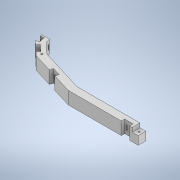
# Autodesk Inventor part: bumper_base_final _원본수정
Saved by Autodesk Inventor 2020 (Build 240168000, 168)
## iProperties
Created: 2022-06-30
Part Number: bumper_base_final _원본수정
Material: 일반
Document SubType Name: Modeling
Designer: samsung
Density: 1 g/cm^3
Appearance: 기본값
Author: samsung
Autodesk Inventor part; units mm, degrees
ref_plane "YZ Plane" through (0, 0, 0) normal (1, 0, 0) x (0, 1, 0)
ref_plane "XZ Plane" through (0, 0, 0) normal (0, 1, 0) x (-1, 0, 0)
ref_plane "XY Plane" through (0, 0, 0) normal (0, 0, 1) x (1, 0, 0)
sketch "스케치1" plane through (0, 0, 0) normal (0, 1, 0) x (-1, 0, 0)
  line L0 (-417.5, 136.0278) -> (167.5, 136.0278)
  arc A0 (156.6099, 73.7155) -> (-406.6899, 73.6783) centre (-125, -531.4722) ccw
  arc A1 (148.4052, 66.4876) -> (-398.3844, 66.4971) centre (-125, -531.4722) ccw
  line L1 (143.8982, 68.5278) -> (-85, 68.5278)
  line L2 (-165, 68.5278) -> (-393.8982, 68.5278)
  line L3 (-125, -531.4722) -> (-125, 1435.9267)
  circle A2 centre (-125, -531.4722) radius 1967.3989
  line L4 (-125, 111.6599) -> (-436.953, 1411.0375)
  line L5 (-125, 111.6599) -> (186.953, 1411.0375)
  line L6 (-417.5444, 28.5399) -> (-406.6899, 73.6783)
  line L7 (-407.5098, 28.5399) -> (-398.3801, 66.5058)
  arc A3 (1441.9544, 38.2515) -> (-1691.7763, 38.7413) centre (-125, -531.4722) ccw
  line L8 (-371.3038, 78.1512) -> (-261.7019, 111.6599)
  line L9 (-261.7019, 111.6599) -> (11.7019, 111.6599)
  line L10 (-316.5029, 94.9056) -> (-320.1581, 106.8613)
  line L11 (-316.5029, 94.9056) -> (-397.3646, 1416.9826)
  line L12 (-316.5029, 94.9056) -> (-988.7616, 1236.1743)
  line L13 (-398.3844, 66.4971) -> (-125, -531.4722)
  line L14 (-407.5098, 28.5399) -> (-405.1717, 38.2627)
  line L15 (-405.1717, 38.2627) -> (-414.6578, 40.5439)
  line L16 (-405.1717, 38.2627) -> (-1671.8283, 684.2501)
  line L17 (-405.1717, 38.2627) -> (-2007.9181, 38.8589)
  line L18 (-405.1717, 38.2627) -> (-402.8337, 47.9856)
  line L19 (-402.8337, 47.9856) -> (-371.3038, 78.1512)
  line L20 (-387.0687, 63.0684) -> (-400.1089, 76.6983)
  line L21 (-387.0687, 63.0684) -> (-1557.9022, 816.656)
  line L22 (-387.0687, 63.0684) -> (-1051.9279, 1203.8846)
  line L23 (-125, -531.4722) -> (-261.7019, 111.6599)
  line L24 (-125, -531.4722) -> (11.7019, 111.6599)
  line L25 (-417.5444, 28.5399) -> (-407.5098, 28.5399)
  line L26 (-125, -531.4722) -> (-371.3038, 78.1512)
  line L27 (-125, -531.4722) -> (121.3038, 78.1512)
  line L28 (11.7019, 111.6599) -> (121.3038, 78.1512)
  line L29 (167.4556, 28.5399) -> (156.6099, 73.7155)
  line L30 (157.5156, 28.5399) -> (148.4052, 66.4876)
  line L31 (121.3038, 78.1512) -> (152.8486, 47.9794)
  line L32 (155.1841, 38.2515) -> (1758.102, 38.2515)
  line L33 (155.1841, 38.2515) -> (164.5823, 40.5079)
  line L34 (157.5156, 28.5399) -> (167.4556, 28.5399)
  line L35 (155.1841, 38.2515) -> (1422.1711, 683.8137)
  line L36 (66.5029, 94.9056) -> (70.1581, 106.8613)
  line L37 (66.5029, 94.9056) -> (738.7616, 1236.1743)
  line L38 (66.5029, 94.9056) -> (147.3646, 1416.9826)
  line L39 (137.0762, 63.0653) -> (150.1137, 76.6961)
  line L40 (137.0762, 63.0653) -> (801.7772, 1203.965)
  line L41 (137.0762, 63.0653) -> (1307.7755, 816.7906)
  line L42 (-125, -531.4722) -> (148.4052, 66.4876)
  line L43 (-259.0118, 93.6599) -> (9.0118, 93.6599)
  line L44 (111.9521, 62.1879) -> (136.5817, 38.6304)
  line L45 (9.0118, 93.6599) -> (111.9521, 62.1879)
  line L46 (-361.9509, 62.1883) -> (-386.641, 38.5664)
  line L47 (-387.0049, 38.256) -> (-387.0101, 38.2515)
  line L48 (-388.9967, 28.5399) -> (-386.569, 38.6353)
  line L49 (-361.9509, 62.1883) -> (-259.0118, 93.6599)
  line L50 (-407.5098, 28.5399) -> (-388.9967, 28.5399)
  line L51 (136.5817, 38.6304) -> (139.0042, 28.5399)
  line L52 (157.5156, 28.5399) -> (139.0042, 28.5399)
  line L53 (-125, 111.6599) -> (-155, 111.6599)
  line L54 (-155, 111.6599) -> (-155, 93.6599)
  line L55 (-155, 93.6599) -> (-125, 93.6599)
  line L56 (-125, 93.6599) -> (-125, 111.6599)
  point P0 (0, 0)
  point P1 (0, 0)
  point P2 (143.8982, 61.5)
  point P3 (-393.8982, 61.5)
  point P4 (-417.5, 21.5)
  point P5 (-165, 0)
  point P6 (-85, 0)
  point P7 (-85, 12.4229)
  point P8 (167.5, 12.4229)
  point P9 (-393.8982, -388.5)
  point P10 (-165, -388.5)
  point P11 (167.5, -327)
  point P12 (-417.5, -327)
  point P13 (-85, -388.5)
  point P14 (143.8982, -388.5)
  point P15 (162, 21.5)
  point P16 (162, 12.4229)
  point P17 (167.5, 21.5)
  point P18 (-125, 0)
  point P19 (-125, 136.0278)
  point P20 (-125, 136.0278)
  point P21 (-125, 93.6599)
  point P22 (-155, 111.6599)
  dimension "d12" = 657.5
  dimension "d13" = 667.5
  dimension "d15" = 585
  dimension "d25" = 1299.8989
  dimension "d30" = 13.5
  dimension "d31" = 13.5
  dimension "d39" = 999.8126
  dimension "d45" = 13.5
  dimension "d46" = 13.5
  dimension "d50" = 10
  dimension "d51" = 13.5
  dimension "d52" = 13.5
  dimension "d53" = 10
  dimension "d54" = 13.5
  dimension "d55" = 13.5
  dimension "d56" = 12
  dimension "d57" = 12
  dimension "d60" = 10
  dimension "d65" = 13.5
  dimension "d66" = 13.5
  dimension "d68" = 13.5
  dimension "d69" = 13.5
  dimension "d70" = 13.5
  dimension "d71" = 13.5
  dimension "d72" = 10
  dimension "d81" = 18
  dimension "d83" = 18
  dimension "d84" = 18
  dimension "d85" = 18
  dimension "d86" = 18
  dimension "d126" = 30
  constraints: 114 end point, 17 point on circle, 14 point on line, 9 parallel, 8 horizontal, 7 perpendicular, 6 midpoint, 3 centre point, 1 coincident, 1 tangent, 18 other
  measures "d12" radius of A1
  measures "d13" radius of A0
  measures "d15" distance of L29.start L6.start
  measures "d30" angle of L4 L3
  measures "d31" angle of L5 L3
  measures "d39" radial gap between concentric circles of A0 A3
  measures "d45" angle of L10 L11
  measures "d46" angle of L12 L10
  measures "d50" distance of L7.start L14.end
  measures "d51" angle of L16 L15
  measures "d52" angle of L17 L15
  measures "d53" distance of L14.end L18.end
  measures "d54" angle of L20 L22
  measures "d55" angle of L20 L21
  measures "d56" angle of L3 L23
  measures "d57" angle of L24 L3
  measures "d60" angle of L26 L23
  measures "d65" angle of L33 L32
  measures "d66" angle of L35 L33
  measures "d68" angle of L37 L36
  measures "d69" angle of L36 L38
  measures "d70" angle of L40 L39
  measures "d71" angle of L41 L39
  measures "d72" angle of L27 L24
  measures "d81" distance between parallel lines of L9 L43
  measures "d83" distance between parallel lines of L31 L44
  measures "d84" distance between parallel lines of L19 L46
  measures "d85" distance between parallel lines of L14 L48
  measures "d86" distance between parallel lines of L30 L51
  measures "d126" distance of L54.end L55.end
extrude "돌출1" add sketch "스케치1" against normal blind 30 contours L9 L24 L43 L3 | L3 L43 L54 L9 | L28 L27 L1 L45 L43 L24 | L44 L45 L1 L27 | L27 L1 L31 L42 L44 | L42 L31 L30 L52 L51 L44 | L31 L1 L27
sketch "스케치2" plane through (-157.5156, -30, 28.5399) normal (-0.9723699, 0, 0.2334454) x (0.2334454, 0, 0.9723699)
  line L0 (4.3214, 30) -> (4.3214, 0) projected
  line L1 (19.9919, 30) -> (56.694, 30) projected
  line L2 (19.9919, 0) -> (0, 0) projected
  line L3 (19.9919, 30) -> (4.9919, 30)
  line L4 (4.9919, 30) -> (4.9919, 0)
  line L5 (4.9919, 0) -> (19.9919, 0)
  line L6 (19.9919, 0) -> (19.9919, 30)
  point P0 (19.9919, 0)
  dimension "d89" = 15
  constraints: 8 end point, 2 parallel, 1 horizontal, 1 perpendicular, 1 point on line
  measures "d89" distance of L5.end L4.end
extrude "돌출2" cut sketch "스케치2" against normal blind 8
sketch "스케치3" plane through (-149.7367, -30, 26.6724) normal (-0.9723699, 0, 0.2334454) x (0.2334454, 0, 0.9723699)
  line L0 (4.9919, 0) -> (4.9919, 30) projected
  line L1 (19.9919, 0) -> (4.9919, 0) projected
  line L2 (19.9919, 30) -> (19.9919, 0) projected
  line L3 (4.9919, 30) -> (19.9919, 30) projected
  line L4 (18.7419, 20.5) -> (16.2419, 20.5)
  line L5 (16.2419, 20.5) -> (16.2419, 9.5)
  line L6 (16.2419, 9.5) -> (18.7419, 9.5)
  line L7 (18.7419, 9.5) -> (18.7419, 20.5)
  line L8 (18.7419, 20.5) -> (16.2419, 9.5) construction
  line L9 (16.2419, 20.5) -> (18.7419, 9.5) construction
  line L10 (6.2419, 20.5) -> (8.7419, 20.5)
  line L11 (8.7419, 20.5) -> (8.7419, 9.5)
  line L12 (8.7419, 9.5) -> (6.2419, 9.5)
  line L13 (6.2419, 9.5) -> (6.2419, 20.5)
  line L14 (6.2419, 20.5) -> (8.7419, 9.5) construction
  line L15 (8.7419, 20.5) -> (6.2419, 9.5) construction
  point P0 (12.4919, 20.5)
  point P1 (12.4919, 30)
  point P2 (19.9919, 15)
  point P3 (17.4919, 15)
  point P4 (7.4919, 15)
  dimension "d94" = 2.5
  dimension "d95" = 2.5
  dimension "d96" = 3.75
  dimension "d97" = 3.75
  dimension "d98" = 9.5
  dimension "d99" = 9.5
  dimension "d100" = 11
  constraints: 24 end point, 6 midpoint, 4 parallel, 2 horizontal, 2 perpendicular, 1 horizontal alignment, 1 vertical alignment
  measures "d94" distance of L6.end L5.end
  measures "d95" distance of L11.end L12.end
  measures "d96" distance from line of point (12.492, 20.5) L5
  measures "d97" distance from line of L11 point (12.492, 20.5)
  measures "d98" distance between parallel lines of L3 L4
  measures "d99" distance between parallel lines of L3 L10
  measures "d100" distance of L10.end L11.end
extrude "돌출3" cut sketch "스케치3" against normal blind 10 contours L7 L6 L5 L4 | L10 L11 L12 L13
sketch "스케치5" plane through (-121.3038, -30, 78.1512) normal (-0.6912048, 0, 0.7226589) x (0.7226589, 0, 0.6912048)
  line L0 (-43.651, 30) -> (0, 30) projected
  line L1 (-43.651, 30) -> (-43.651, 0) projected
  line L2 (0, 0) -> (-43.651, 0) projected
  line L3 (0, 30) -> (0, 0) projected
  line L4 (-38.3577, 0) -> (-4.2758, 0) projected
  line L5 (-31.8255, 30) -> (-11.8255, 30)
  line L6 (-11.8255, 30) -> (-11.8255, 0)
  line L7 (-11.8255, 0) -> (-31.8255, 0)
  line L8 (-31.8255, 0) -> (-31.8255, 30)
  line L9 (-31.8255, 30) -> (-11.8255, 0) construction
  line L10 (-11.8255, 30) -> (-31.8255, 0) construction
  point P0 (33.6428, 30)
  point P1 (-21.8255, 15)
  point P2 (-31.8255, 30)
  point P3 (-31.8255, 0)
  dimension "d107" = 20
  constraints: 12 end point, 2 midpoint, 2 parallel, 1 horizontal, 1 perpendicular, 1 point on line
  measures "d107" distance of L6.end L7.end
extrude "돌출4" cut sketch "스케치5" against normal blind 8 contours L0 L6 L2 L8
sketch "스케치6" plane through (-115.7742, -30, 72.37) normal (-0.6912048, 0, 0.7226589) x (0.7226589, 0, 0.6912048)
  line L0 (-11.8255, 0) -> (-31.8255, 0) projected
  line L1 (-11.8255, 30) -> (-11.8255, 0) projected
  line L2 (-31.8255, 30) -> (-11.8255, 30) projected
  line L3 (-31.8255, 0) -> (-31.8255, 30) projected
  line L4 (-26.8255, 20.5) -> (-16.8255, 9.5) construction
  line L5 (-16.8255, 20.5) -> (-26.8255, 9.5) construction
  line L6 (-15.5755, 20.5) -> (-18.0755, 20.5)
  line L7 (-18.0755, 20.5) -> (-18.0755, 9.5)
  line L8 (-18.0755, 9.5) -> (-15.5755, 9.5)
  line L9 (-15.5755, 9.5) -> (-15.5755, 20.5)
  line L10 (-15.5755, 20.5) -> (-18.0755, 9.5) construction
  line L11 (-18.0755, 20.5) -> (-15.5755, 9.5) construction
  line L12 (-28.0755, 20.5) -> (-25.5755, 20.5)
  line L13 (-25.5755, 20.5) -> (-25.5755, 9.5)
  line L14 (-25.5755, 9.5) -> (-28.0755, 9.5)
  line L15 (-28.0755, 9.5) -> (-28.0755, 20.5)
  line L16 (-28.0755, 20.5) -> (-25.5755, 9.5) construction
  line L17 (-25.5755, 20.5) -> (-28.0755, 9.5) construction
  point P0 (33.6428, 30)
  point P1 (-21.8255, 15)
  point P2 (-16.8255, 15)
  point P3 (-26.8255, 15)
  dimension "d110" = 10
  dimension "d111" = 11
  dimension "d112" = 2.5
  dimension "d113" = 2.5
  constraints: 28 end point, 6 midpoint, 4 parallel, 2 horizontal, 2 perpendicular
  measures "d110" distance of L4.end L5.end
  measures "d111" distance of L5.start L4.end
  measures "d112" distance of L8.end L7.end
  measures "d113" distance of L13.end L14.end
extrude "돌출5" cut sketch "스케치6" against normal blind 10 contours L9 L8 L7 L6 | L12 L13 L14 L15
sketch "스케치7" plane through (-121.3038, -30, 78.1512) normal (-0.2923717, 0, 0.9563048) x (0.9563048, 0, 0.2923717)
  line L0 (0, 30) -> (114.6098, 30) projected
  line L1 (0, 30) -> (0, 0) projected
  line L2 (114.6098, 0) -> (0, 0) projected
  line L3 (114.6098, 30) -> (114.6098, 0) projected
  line L4 (4.2758, 0) -> (111.9197, 0) projected
  line L5 (47.3049, 30) -> (67.3049, 30)
  line L6 (67.3049, 30) -> (67.3049, 0)
  line L7 (67.3049, 0) -> (47.3049, 0)
  line L8 (47.3049, 0) -> (47.3049, 30)
  line L9 (47.3049, 30) -> (67.3049, 0) construction
  line L10 (67.3049, 30) -> (47.3049, 0) construction
  point P0 (93.1542, 30)
  point P1 (57.3049, 15)
  point P2 (47.3049, 30)
  point P3 (47.3049, 0)
  dimension "d116" = 20
  dimension "d117" = 30
  constraints: 12 end point, 2 midpoint, 2 parallel, 1 horizontal, 1 perpendicular, 1 point on line
  measures "d116" distance of L6.end L7.end
  measures "d117" distance of L5.end L6.end
extrude "돌출6" cut sketch "스케치7" against normal blind 8 contours L0 L6 L2 L8
sketch "스케치8" plane through (-118.9649, -30, 70.5008) normal (-0.2923717, 0, 0.9563048) x (0.9563048, 0, 0.2923717)
  line L0 (47.3049, 0) -> (47.3049, 30) projected
  line L1 (67.3049, 0) -> (47.3049, 0) projected
  line L2 (67.3049, 30) -> (67.3049, 0) projected
  line L3 (47.3049, 30) -> (67.3049, 30) projected
  line L4 (52.3049, 20.5) -> (62.3049, 9.5) construction
  line L5 (62.3049, 20.5) -> (52.3049, 9.5) construction
  line L6 (51.0549, 20.5) -> (53.5549, 20.5)
  line L7 (53.5549, 20.5) -> (53.5549, 9.5)
  line L8 (53.5549, 9.5) -> (51.0549, 9.5)
  line L9 (51.0549, 9.5) -> (51.0549, 20.5)
  line L10 (51.0549, 20.5) -> (53.5549, 9.5) construction
  line L11 (53.5549, 20.5) -> (51.0549, 9.5) construction
  line L12 (63.5549, 20.5) -> (61.0549, 20.5)
  line L13 (61.0549, 20.5) -> (61.0549, 9.5)
  line L14 (61.0549, 9.5) -> (63.5549, 9.5)
  line L15 (63.5549, 9.5) -> (63.5549, 20.5)
  line L16 (63.5549, 20.5) -> (61.0549, 9.5) construction
  line L17 (61.0549, 20.5) -> (63.5549, 9.5) construction
  point P0 (93.1542, 30)
  point P1 (57.3049, 15)
  point P2 (52.3049, 15)
  point P3 (62.3049, 15)
  dimension "d120" = 10
  dimension "d121" = 11
  dimension "d122" = 2.5
  dimension "d123" = 2.5
  constraints: 28 end point, 6 midpoint, 4 parallel, 2 horizontal, 2 perpendicular
  measures "d120" distance of L4.end L5.end
  measures "d121" distance of L5.start L4.end
  measures "d122" distance of L7.end L8.end
  measures "d123" distance of L14.end L13.end
extrude "돌출7" cut sketch "스케치8" against normal blind 10 contours L6 L7 L8 L9 | L15 L14 L13 L12
sketch "스케치9" plane through (-11.7019, 0, 111.6599) normal (0, 0, 1) x (1, 0, 0)
  line L0 (0, 0) -> (166.7019, 0) projected
  line L1 (0, 0) -> (0, -30) projected
  line L2 (166.7019, -30) -> (0, -30) projected
  line L3 (166.7019, 0) -> (166.7019, -30) projected
  line L4 (166.7019, 0) -> (2.6901, 0) projected
  line L5 (2.6901, -30) -> (166.7019, -30) projected
  line L6 (146.7019, 0) -> (126.7019, 0)
  line L7 (126.7019, 0) -> (126.7019, -30)
  line L8 (126.7019, -30) -> (146.7019, -30)
  line L9 (146.7019, -30) -> (146.7019, 0)
  point P0 (11.7019, 0)
  point P1 (146.7019, -30)
  point P2 (126.7019, 0)
  point P3 (126.7019, -30)
  dimension "d127" = 20
  dimension "d128" = 20
  constraints: 8 end point, 2 parallel, 2 point on line, 1 horizontal, 1 perpendicular
  measures "d127" distance of L8.end L7.end
  measures "d128" distance between parallel lines of L9 L3
extrude "돌출8" cut sketch "스케치9" against normal blind 8 contours L0 L9 L2 L7
sketch "스케치10" plane through (-11.7019, 0, 103.6599) normal (0, 0, 1) x (1, 0, 0)
  line L0 (126.7019, -30) -> (126.7019, 0) projected
  line L1 (146.7019, -30) -> (126.7019, -30) projected
  line L2 (146.7019, 0) -> (146.7019, -30) projected
  line L3 (126.7019, 0) -> (146.7019, 0) projected
  line L4 (131.7019, -9.5) -> (141.7019, -20.5) construction
  line L5 (141.7019, -9.5) -> (131.7019, -20.5) construction
  line L6 (140.4519, -9.5) -> (142.9519, -9.5)
  line L7 (142.9519, -9.5) -> (142.9519, -20.5)
  line L8 (142.9519, -20.5) -> (140.4519, -20.5)
  line L9 (140.4519, -20.5) -> (140.4519, -9.5)
  line L10 (140.4519, -9.5) -> (142.9519, -20.5) construction
  line L11 (142.9519, -9.5) -> (140.4519, -20.5) construction
  line L12 (130.4519, -9.5) -> (132.9519, -9.5)
  line L13 (132.9519, -9.5) -> (132.9519, -20.5)
  line L14 (132.9519, -20.5) -> (130.4519, -20.5)
  line L15 (130.4519, -20.5) -> (130.4519, -9.5)
  line L16 (130.4519, -9.5) -> (132.9519, -20.5) construction
  line L17 (132.9519, -9.5) -> (130.4519, -20.5) construction
  line L18 (126.7019, 0) -> (146.7019, 0) projected
  point P0 (11.7019, 0)
  point P1 (136.7019, -15)
  point P2 (141.7019, -15)
  point P3 (131.7019, -15)
  point P4 (136.7019, -15)
  point P5 (136.7019, 0)
  point P6 (136.7019, -15)
  point P7 (136.7019, 0)
  point P8 (126.7019, -15)
  point P9 (146.7019, -15)
  dimension "d131" = 10
  dimension "d132" = 11
  dimension "d133" = 2.5
  dimension "d134" = 2.5
  constraints: 28 end point, 16 midpoint, 4 parallel, 2 horizontal, 2 horizontal alignment, 2 perpendicular, 2 vertical alignment
  measures "d131" distance of L5.end L4.end
  measures "d132" distance of L5.start L4.end
  measures "d133" distance of L7.end L8.end
  measures "d134" distance of L13.end L14.end
extrude "돌출9" cut sketch "스케치10" against normal blind 10 contours L6 L7 L8 L9 | L12 L13 L14 L15
sketch "스케치11" plane through (155, 0, 111.6599) normal (1, 0, 0) x (0, 0, -1)
  line L0 (0, 0) -> (18, 0) projected
  line L1 (0, 0) -> (0, -30) projected
  line L2 (18, -30) -> (0, -30) projected
  line L3 (18, 0) -> (18, -30) projected
  line L4 (18, 0) -> (18, -30) projected
  line L5 (18, -10) -> (0, -10)
  point P0 (111.6599, 0)
  point P1 (18, -10)
  point P2 (0, -10)
  dimension "d139" = 10
  constraints: 2 end point
  measures "d139" distance between parallel lines of L0 L5
extrude "돌출10" cut sketch "스케치11" against normal blind 14 contours L0 L3 L5 L1
sketch "스케치12" plane through (0, -30, 0) normal (0, -1, 0) x (1, 0, 0)
  line L0 (-157.5156, 28.5399) -> (-139.0042, 28.5399) projected
  point P0 (0, 0)
  point P1 (-117.5156, 68.5399)
  dimension "d149" = 40
  dimension "d150" = 40
  measures "d149" distance from line of point (-117.516, 68.54) L0
  measures "d150" horizontal distance of point (-117.516, 68.54) L0.start
hole "구멍1" at (-117.5156, -30, 68.5399) direction (0, 1, 0) diameter 4.2 end through all counterbore diameter 8 counterbore depth 15
sketch "스케치13" plane through (0, -30, 0) normal (0, -1, 0) x (1, 0, 0)
  line L0 (155, 93.6599) -> (155, 111.6599) projected
  line L1 (-9.0118, 93.6599) -> (155, 93.6599) projected
  line L2 (115, 103.6599) -> (135, 103.6599) projected
  point P0 (0, 0)
  point P1 (148, 102.6599)
  dimension "d151" = 7
  dimension "d159" = 9
  measures "d151" distance from line of L0 point (148, 102.66)
  measures "d159" distance from line of L1 point (148, 102.66)
hole "구멍2" at (148, -30, 102.6599) direction (0, 1, 0) diameter 4.2 end through all counterbore diameter 8 counterbore depth 15
equation "\"d46\" = d45"
equation "\"d57\" = d56"
equation "\"d72\" = d60"
equation "\"d61\" = d60"
